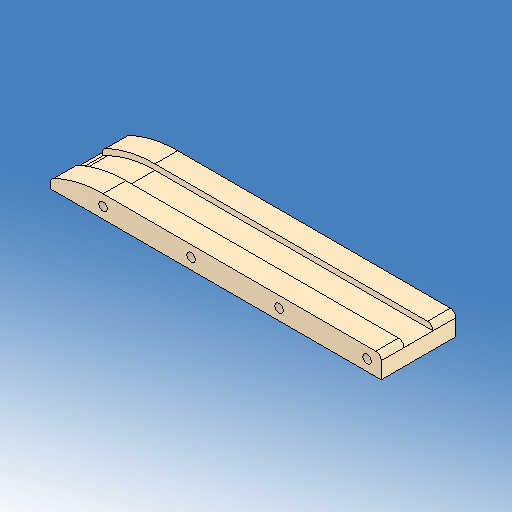
# Autodesk Inventor part: chain guide
Saved by Autodesk Inventor 2025 (Build 290162000, 162)
## iProperties
Created: 2023-03-01
Part Number: chain guide
Material: Polyethylene, High Density
Document SubType Name: Modeling
Designer: ralph
Density: 0.952 g/cm^3
Appearance: Smooth - Off-White
Author: ralph
Autodesk Inventor part; units mm, degrees
(part 1 of 2)
ref_plane "Work Plane1" through (161.724971, -21.836185, 0) normal (0, 0, 1) x (-0.4541702, 0.8909149, 0)
ref_plane "Work Plane2" through (-185.342071, -221.252054, 43.0784) normal (0, 0, -1) x (-0.1993348, 0.9799314, 0)
sketch "Sketch1" plane through (161.724971, -21.836185, 0) normal (0, 0, 1) x (-0.4541702, 0.8909149, 0)
  circle A0 centre (-25.19799, 87.680503) radius 3.175
  line L0 (-137.960154, 56.932811) -> (35.815717, 235.351647)
  line L1 (82.547855, 91.780244) -> (42.733083, 68.543644)
  line L2 (134.381301, 156.187054) -> (107.829785, 115.760327)
  line L3 (-111.140721, 21.588661) -> (-101.506151, 29.862833)
  line L4 (-105.643304, 34.680133) -> (-115.277874, 26.405961)
  line L5 (-3.594311, 192.040273) -> (-4.303422, 192.730924)
  line L6 (-3.594311, 192.040273) -> (-10.222625, 185.234864)
  line L7 (-10.931735, 185.925514) -> (-10.222625, 185.234864)
  arc A1 (2.942016, 134.774843) -> (-78.867042, 82.739265) centre (-35.469099, 104.836969) ccw
  line L8 (2.942016, 134.774843) -> (32.675099, 96.626481)
  arc A2 (44.414913, 71.120558) -> (32.675099, 96.626481) centre (-15.752877, 58.8814) ccw
  line L9 (44.414913, 71.120558) -> (83.682207, -121.91774)
  arc A3 (34.145903, -139.208204) -> (83.682207, -121.91774) centre (57.738523, -127.19513) ccw
  line L10 (34.145903, -139.208204) -> (-78.867042, 82.739265)
  line L11 (86.79349, -121.284852) -> (47.526196, 71.753446)
  arc A4 (47.526196, 71.753446) -> (35.179314, 98.578283) centre (-15.752877, 58.8814) ccw
  line L12 (35.179314, 98.578283) -> (5.446231, 136.726645)
  arc A5 (5.446231, 136.726645) -> (-81.696374, 81.298604) centre (-35.469099, 104.836969) ccw
  line L13 (-81.696374, 81.298604) -> (31.316571, -140.648865)
  arc A6 (31.316571, -140.648865) -> (86.79349, -121.284852) centre (57.738523, -127.19513) ccw
  line L14 (74.34836, -123.816404) -> (35.081066, 69.221894)
  arc A7 (35.081066, 69.221894) -> (25.162453, 90.771076) centre (-15.752877, 58.8814) ccw
  line L15 (25.162453, 90.771076) -> (-4.57063, 128.919438)
  arc A8 (-4.57063, 128.919438) -> (-70.379046, 87.061249) centre (-35.469099, 104.836969) ccw
  line L16 (-70.379046, 87.061249) -> (42.6339, -134.88622)
  arc A9 (42.6339, -134.88622) -> (74.34836, -123.816404) centre (57.738523, -127.19513) ccw
  arc A10 (5.840596, 137.034015) -> (-82.141938, 81.071728) centre (-35.469099, 104.836969) ccw
  line L17 (5.840596, 137.034015) -> (35.573679, 98.885654)
  arc A11 (48.016161, 71.853114) -> (35.573679, 98.885654) centre (-15.752877, 58.8814) ccw
  line L18 (48.016161, 71.853114) -> (87.283455, -121.185185)
  arc A12 (30.871007, -140.875741) -> (87.283455, -121.185185) centre (57.738523, -127.19513) ccw
  line L19 (30.871007, -140.875741) -> (-82.141938, 81.071728)
  line L20 (35.081066, 69.221894) -> (26.965843, 109.116392)
  circle A13 centre (57.738523, -127.19513) radius 44.45
  line L21 (76.564874, -86.928878) -> (65.823198, -81.906643)
  line L22 (5.091971, 163.504868) -> (21.707035, 97.430996)
  line L23 (16.959788, 93.955303) -> (-30.179917, 123.063587)
  line L24 (-32.869192, 137.518787) -> (-4.591446, 166.552061)
  line L25 (29.816468, 96.427864) -> (15.424243, 153.662068)
  line L26 (20.79343, 156.635425) -> (60.850023, 114.922703)
  line L27 (59.720131, 100.498003) -> (42.266373, 90.311684)
  line L28 (16.752459, 188.466235) -> (29.554478, 201.6103)
  line L29 (102.791645, 142.788647) -> (91.891787, 126.192776)
  line L30 (66.346153, 120.200561) -> (40.797068, 146.805966)
  line L31 (-106.606458, 61.811399) -> (-103.834749, 64.657164)
  line L32 (-88.173268, 62.778772) -> (-84.305135, 57.816691)
  line L33 (-71.902397, 23.680787) -> (-75.267331, 21.716952)
  line L34 (-82.428573, 45.397297) -> (-80.279259, 47.243129)
  line L35 (-75.706636, 46.78645) -> (-69.919657, 39.362855)
  line L36 (41.018546, 151.413723) -> (46.086473, 155.76606)
  line L37 (41.121889, 161.54682) -> (35.464526, 156.688275)
  line L38 (31.105895, 156.897817) -> (17.932591, 170.615767)
  line L39 (-84.740604, 53.45607) -> (-87.393157, 51.178057)
  arc A14 (19.642871, 91.662594) -> (21.445924, 90.856947) centre (24.92977, 101.074326) ccw
  arc A15 (23.578481, 87.516275) -> (21.445924, 90.856947) centre (20.421264, 87.851835) ccw
  arc A16 (23.578481, 87.516275) -> (24.03183, 82.566279) centre (36.191661, 86.175702) ccw
  arc A17 (22.700522, 78.989189) -> (24.03183, 82.566279) centre (20.98809, 81.662801) ccw
  line L40 (22.700522, 78.989189) -> (6.045724, 68.321892)
  arc A18 (2.215102, 68.630362) -> (6.045724, 68.321892) centre (4.333292, 70.995504) ccw
  arc A19 (2.215102, 68.630362) -> (-6.080111, 71.872214) centre (-6.267606, 59.158683) ccw
  arc A20 (-8.905438, 73.693574) -> (-6.080111, 71.872214) centre (-6.033293, 75.046869) ccw
  line L41 (-8.905438, 73.693574) -> (-12.804922, 81.969586)
  arc A21 (-12.985819, 84.194406) -> (-12.804922, 81.969586) centre (-9.932777, 83.322881) ccw
  arc A22 (-12.985819, 84.194406) -> (-20.111454, 99.31739) centre (-25.19799, 87.680503) ccw
  arc A23 (-21.711965, 100.873317) -> (-20.111454, 99.31739) centre (-18.839819, 102.226612) ccw
  line L42 (-21.711965, 100.873317) -> (-28.578282, 115.445944)
  arc A24 (-26.364724, 117.50667) -> (-28.578282, 115.445944) centre (-27.142209, 116.122592) ccw
  line L43 (-26.364724, 117.50667) -> (19.642871, 91.662594)
  line L44 (-65.60794, 77.010503) -> (-80.772151, 80.874337)
  line L45 (-82.490843, 86.571338) -> (-54.213097, 115.604612)
  line L46 (-42.284096, 112.695685) -> (-42.24754, 112.608973)
  line L47 (-99.979245, 13.668511) -> (-98.035437, 10.337963)
  line L48 (118.443303, 166.619502) -> (116.943486, 164.335916)
  line L49 (-124.328477, 43.615881) -> (-123.070102, 44.907878)
  line L50 (-120.825239, 44.937466) -> (-116.194419, 40.427197)
  line L51 (-43.104595, 108.966969) -> (-65.061673, 90.110222)
  line L52 (-65.401739, 85.633029) -> (-62.415382, 82.155716)
  ellipse E0 centre (81.305166, 191.046395) end of major axis (135.808144, 158.463034) minor radius 63.499313 (134.381301, 156.187054) -> (35.815717, 235.351647) ccw
  ellipse E1 centre (44.138423, 157.591537) end of major axis (-21.265151, 196.691569) minor radius 76.199176 (82.547855, 91.780244) -> (107.829785, 115.760327) ccw
  ellipse E2 centre (-113.209297, 23.997311) end of major axis (-115.934446, 25.626479) minor radius 3.174966 (-115.277874, 26.405961) -> (-111.140721, 21.588661) ccw
  ellipse E3 centre (-103.574727, 32.271483) end of major axis (-106.299876, 33.900651) minor radius 3.174966 (-101.506151, 29.862833) -> (-105.643304, 34.680133) ccw
  ellipse E4 centre (5.31041, 178.259198) end of major axis (-5.590186, 184.77587) minor radius 12.699863 (-0.791497, 167.121278) -> (2.672353, 165.836334) ccw
  ellipse E5 centre (2.012839, 162.730619) end of major axis (-0.71231, 164.359787) minor radius 3.174966 (5.091971, 163.504868) -> (2.672353, 165.836334) ccw
  ellipse E6 centre (18.627903, 96.656747) end of major axis (21.353052, 95.027579) minor radius 3.174966 (16.959788, 93.955303) -> (21.707035, 97.430996) ccw
  ellipse E7 centre (-28.511802, 125.76503) end of major axis (-25.786653, 124.135862) minor radius 3.174966 (-31.67169, 126.074374) -> (-30.179917, 123.063587) ccw
  ellipse E8 centre (-44.311242, 127.311749) end of major axis (-55.211837, 133.828421) minor radius 12.699863 (-31.67169, 126.074374) -> (-33.338024, 133.705169) ccw
  ellipse E9 centre (-30.59472, 135.303524) end of major axis (-27.869571, 133.674356) minor radius 3.174966 (-32.869192, 137.518787) -> (-33.338024, 133.705169) ccw
  ellipse E10 centre (-2.316974, 164.336798) end of major axis (-5.042123, 165.965966) minor radius 3.174966 (-0.791497, 167.121278) -> (-4.591446, 166.552061) ccw
  ellipse E11 centre (32.8956, 97.202113) end of major axis (35.620749, 95.572945) minor radius 3.174966 (29.816468, 96.427864) -> (32.236086, 94.096397) ccw
  ellipse E12 centre (18.503375, 154.436317) end of major axis (15.778226, 156.065485) minor radius 3.174966 (20.79343, 156.635425) -> (15.424243, 153.662068) ccw
  ellipse E13 centre (58.559969, 112.723596) end of major axis (55.83482, 114.352764) minor radius 3.174966 (61.542416, 111.634731) -> (60.850023, 114.922703) ccw
  ellipse E14 centre (73.472205, 107.279273) end of major axis (62.571609, 113.795945) minor radius 12.699863 (61.542416, 111.634731) -> (61.190231, 104.047967) ccw
  ellipse E15 centre (58.119738, 103.240141) end of major axis (60.844887, 101.610973) minor radius 3.174966 (59.720131, 100.498003) -> (61.190231, 104.047967) ccw
  ellipse E16 centre (40.66598, 93.053821) end of major axis (43.391128, 91.424653) minor radius 3.174966 (38.452389, 90.777764) -> (42.266373, 90.311684) ccw
  ellipse E17 centre (20.222646, 172.814875) end of major axis (22.947795, 171.185707) minor radius 3.174966 (17.240198, 173.903739) -> (17.932591, 170.615767) ccw
  ellipse E18 centre (5.31041, 178.259198) end of major axis (-5.590186, 184.77587) minor radius 12.699863 (17.240198, 173.903739) -> (16.283627, 184.652618) ccw
  ellipse E19 centre (19.026932, 186.250973) end of major axis (21.752081, 184.621805) minor radius 3.174966 (16.752459, 188.466235) -> (16.283627, 184.652618) ccw
  ellipse E20 centre (31.82895, 199.395037) end of major axis (29.103801, 201.024205) minor radius 3.174966 (34.959397, 198.865037) -> (29.554478, 201.6103) ccw
  ellipse E21 centre (81.290008, 191.021041) end of major axis (40.957805, 215.132728) minor radius 46.989492 (50.252199, 155.741184) -> (98.944937, 147.473983) ccw
  ellipse E22 centre (100.137838, 144.531614) end of major axis (97.412689, 146.160782) minor radius 3.174966 (102.791645, 142.788647) -> (98.944937, 147.473983) ccw
  ellipse E23 centre (44.123265, 157.566183) end of major axis (-4.929415, 186.891207) minor radius 57.149382 (85.199308, 117.83109) -> (91.891787, 126.192776) ccw
  ellipse E24 centre (82.917305, 120.038595) end of major axis (85.642454, 118.409427) minor radius 3.174966 (81.028285, 117.486731) -> (85.199308, 117.83109) ccw
  ellipse E25 centre (73.472205, 107.279273) end of major axis (62.571609, 113.795945) minor radius 12.699863 (81.028285, 117.486731) -> (69.603407, 119.37559) ccw
  ellipse E26 centre (68.636207, 122.399669) end of major axis (71.361356, 120.770501) minor radius 3.174966 (66.346153, 120.200561) -> (69.603407, 119.37559) ccw
  ellipse E27 centre (-108.40717, 28.109043) end of major axis (-132.93351, 42.771555) minor radius 28.574691 (-80.021668, 24.824085) -> (-83.164714, 41.500687) ccw
  ellipse E28 centre (-104.331986, 59.596136) end of major axis (-101.606837, 57.966968) minor radius 3.174966 (-106.606458, 61.811399) -> (-104.739504, 56.447427) ccw
  ellipse E29 centre (-101.560276, 62.441901) end of major axis (-104.285425, 64.071069) minor radius 3.174966 (-100.034799, 65.226381) -> (-103.834749, 64.657164) ccw
  ellipse E30 centre (-93.932893, 76.3643) end of major axis (-83.032297, 69.847628) minor radius 12.699863 (-100.034799, 65.226381) -> (-91.32843, 63.934301) ccw
  ellipse E31 centre (-90.677314, 60.826801) end of major axis (-93.402463, 62.455969) minor radius 3.174966 (-88.173268, 62.778772) -> (-91.32843, 63.934301) ccw
  ellipse E32 centre (-72.423703, 37.410884) end of major axis (-75.148852, 39.040052) minor radius 3.174966 (-69.569027, 36.021118) -> (-69.919657, 39.362855) ccw
  ellipse E33 centre (-58.150322, 30.462056) end of major axis (-69.050918, 36.978728) minor radius 12.699863 (-69.569027, 36.021118) -> (-70.432296, 27.23075) ccw
  ellipse E34 centre (-73.50279, 26.422924) end of major axis (-70.777641, 24.793756) minor radius 3.174966 (-71.902397, 23.680787) -> (-70.432296, 27.23075) ccw
  ellipse E35 centre (-76.867724, 24.459089) end of major axis (-74.142575, 22.829921) minor radius 3.174966 (-80.021668, 24.824085) -> (-75.267331, 21.716952) ccw
  ellipse E36 centre (-108.40717, 28.109043) end of major axis (-132.93351, 42.771555) minor radius 28.574691 (-91.356277, 51.038941) -> (-104.739504, 56.447427) ccw
  ellipse E37 centre (81.290008, 191.021041) end of major axis (40.957805, 215.132728) minor radius 46.989492 (34.959397, 198.865037) -> (41.726521, 165.668481) ccw
  ellipse E38 centre (-80.359997, 42.988647) end of major axis (-83.085146, 44.617815) minor radius 3.174966 (-82.428573, 45.397297) -> (-83.164714, 41.500687) ccw
  ellipse E39 centre (-78.210682, 44.834479) end of major axis (-80.935831, 46.463647) minor radius 3.174966 (-75.706636, 46.78645) -> (-80.279259, 47.243129) ccw
  ellipse E40 centre (43.087122, 149.005073) end of major axis (45.812271, 147.375905) minor radius 3.174966 (41.018546, 151.413723) -> (40.797068, 146.805966) ccw
  ellipse E41 centre (48.155049, 153.35741) end of major axis (45.4299, 154.986578) minor radius 3.174966 (50.252199, 155.741184) -> (46.086473, 155.76606) ccw
  ellipse E42 centre (33.39595, 159.096925) end of major axis (36.121098, 157.467757) minor radius 3.174966 (31.105895, 156.897817) -> (35.464526, 156.688275) ccw
  ellipse E43 centre (39.053313, 163.95547) end of major axis (36.328164, 165.584638) minor radius 3.174966 (41.121889, 161.54682) -> (41.726521, 165.668481) ccw
  ellipse E44 centre (-86.80918, 55.86472) end of major axis (-89.534329, 57.493888) minor radius 3.174966 (-84.740604, 53.45607) -> (-84.305135, 57.816691) ccw
  ellipse E45 centre (-89.461733, 53.586707) end of major axis (-86.736584, 51.957539) minor radius 3.174966 (-91.356277, 51.038941) -> (-87.393157, 51.178057) ccw
  ellipse E46 centre (-79.988236, 83.951008) end of major axis (-77.263087, 82.32184) minor radius 3.174966 (-82.777167, 82.433666) -> (-80.772151, 80.874337) ccw
  ellipse E47 centre (-93.932893, 76.3643) end of major axis (-104.833488, 82.880972) minor radius 12.699863 (-82.777167, 82.433666) -> (-82.959675, 82.75772) ccw
  ellipse E48 centre (-80.216371, 84.356075) end of major axis (-77.491222, 82.726907) minor radius 3.174966 (-82.490843, 86.571338) -> (-82.959675, 82.75772) ccw
  ellipse E49 centre (-51.938625, 113.38935) end of major axis (-54.663774, 115.018518) minor radius 3.174966 (-50.413148, 116.173829) -> (-54.213097, 115.604612) ccw
  ellipse E50 centre (-44.311242, 127.311749) end of major axis (-33.410646, 120.795077) minor radius 12.699863 (-50.413148, 116.173829) -> (-45.03003, 114.632214) ccw
  ellipse E51 centre (-45.209727, 111.46233) end of major axis (-47.934876, 113.091498) minor radius 3.174966 (-42.284096, 112.695685) -> (-45.03003, 114.632214) ccw
  ellipse E52 centre (69.174216, 230.477557) end of major axis (66.449067, 232.106725) minor radius 3.174966 (71.822052, 228.725533) -> (68.242232, 233.512673) ccw
  ellipse E53 centre (87.709071, 218.213391) end of major axis (71.358177, 227.988399) minor radius 19.049794 (71.822052, 228.725533) -> (69.767585, 224.616929) ccw
  ellipse E54 centre (66.777338, 225.684185) end of major axis (69.502486, 224.055017) minor radius 3.174966 (65.439426, 222.80488) -> (69.767585, 224.616929) ccw
  ellipse E55 centre (57.411955, 205.529045) end of major axis (41.061062, 215.304053) minor radius 19.049794 (65.439426, 222.80488) -> (61.070524, 224.224243) ccw
  ellipse E56 centre (61.680285, 227.340109) end of major axis (64.405434, 225.710941) minor radius 3.174966 (60.171845, 230.133884) -> (61.070524, 224.224243) ccw
  ellipse E57 centre (81.290008, 191.021041) end of major axis (119.442093, 168.212688) minor radius 44.449519 (68.242232, 233.512673) -> (60.171845, 230.133884) ccw
  ellipse E58 centre (115.071482, 214.736161) end of major axis (117.796631, 213.106993) minor radius 3.174966 (114.22345, 211.676543) -> (117.670057, 216.560401) ccw
  ellipse E59 centre (109.13526, 193.318833) end of major axis (92.784366, 203.093841) minor radius 19.049794 (114.22345, 211.676543) -> (109.681031, 212.360856) ccw
  ellipse E60 centre (109.771993, 215.534527) end of major axis (112.497142, 213.905359) minor radius 3.174966 (106.620147, 215.917221) -> (109.681031, 212.360856) ccw
  ellipse E61 centre (87.709071, 218.213391) end of major axis (71.358177, 227.988399) minor radius 19.049794 (106.620147, 215.917221) -> (106.619944, 220.510867) ccw
  ellipse E62 centre (109.771757, 220.89378) end of major axis (107.046608, 222.522948) minor radius 3.174966 (111.96266, 223.191683) -> (106.619944, 220.510867) ccw
  ellipse E63 centre (81.290008, 191.021041) end of major axis (119.442093, 168.212688) minor radius 44.449519 (117.670057, 216.560401) -> (111.96266, 223.191683) ccw
  ellipse E64 centre (-99.406505, 9.537784) end of major axis (-98.043931, 8.7232) minor radius 1.587483 (-98.714147, 8.109225) -> (-98.035437, 10.337963) ccw
  ellipse E65 centre (-108.40717, 28.109043) end of major axis (-127.483212, 39.513219) minor radius 22.22476 (-107.641506, 5.897406) -> (-98.714147, 8.109225) ccw
  ellipse E66 centre (-107.750887, 9.070497) end of major axis (-110.476036, 10.699665) minor radius 3.174966 (-108.8456, 12.050789) -> (-107.641506, 5.897406) ccw
  ellipse E67 centre (-113.224455, 23.971957) end of major axis (-102.323859, 17.455285) minor radius 12.699863 (-108.8456, 12.050789) -> (-104.821996, 14.448914) ccw
  ellipse E68 centre (-102.721381, 12.068153) end of major axis (-99.996232, 10.438985) minor radius 3.174966 (-99.979245, 13.668511) -> (-104.821996, 14.448914) ccw
  ellipse E69 centre (114.28968, 166.078883) end of major axis (117.014829, 164.449715) minor radius 3.174966 (111.116905, 165.9603) -> (116.943486, 164.335916) ccw
  ellipse E70 centre (92.080258, 165.248804) end of major axis (75.729364, 175.023813) minor radius 19.049794 (111.116905, 165.9603) -> (110.359048, 170.613884) ccw
  ellipse E71 centre (113.405514, 171.508064) end of major axis (110.680365, 173.137232) minor radius 3.174966 (112.795477, 174.623888) -> (110.359048, 170.613884) ccw
  ellipse E72 centre (109.13526, 193.318833) end of major axis (92.784366, 203.093841) minor radius 19.049794 (112.795477, 174.623888) -> (117.164254, 176.043554) ccw
  ellipse E73 centre (118.50242, 173.16434) end of major axis (115.777271, 174.793508) minor radius 3.174966 (121.364913, 171.790748) -> (117.164254, 176.043554) ccw
  ellipse E74 centre (81.290008, 191.021041) end of major axis (119.442093, 168.212688) minor radius 44.449519 (118.443303, 166.619502) -> (121.364913, 171.790748) ccw
  ellipse E75 centre (-121.932866, 43.800246) end of major axis (-123.29544, 44.61483) minor radius 1.587483 (-120.825239, 44.937466) -> (-123.070102, 44.907878) ccw
  ellipse E76 centre (-117.302045, 39.289977) end of major axis (-118.66462, 40.104561) minor radius 1.587483 (-116.313726, 38.047651) -> (-116.194419, 40.427197) ccw
  ellipse E77 centre (-108.40717, 28.109043) end of major axis (-119.307765, 34.625715) minor radius 12.699863 (-116.313726, 38.047651) -> (-118.827374, 35.369161) ccw
  ellipse E78 centre (-113.224455, 23.971957) end of major axis (-102.323859, 17.455285) minor radius 12.699863 (-118.827374, 35.369161) -> (-124.347508, 30.101205) ccw
  ellipse E79 centre (-127.128271, 31.633517) end of major axis (-129.85342, 33.262685) minor radius 3.174966 (-130.248455, 32.22093) -> (-124.347508, 30.101205) ccw
  ellipse E80 centre (-108.40717, 28.109043) end of major axis (-127.483212, 39.513219) minor radius 22.22476 (-124.328477, 43.615881) -> (-130.248455, 32.22093) ccw
  ellipse E81 centre (29.598029, 81.673534) end of major axis (18.697433, 88.190206) minor radius 12.699863 (38.452389, 90.777764) -> (32.236086, 94.096397) ccw
  ellipse E82 centre (-62.993097, 87.701572) end of major axis (-60.267948, 86.072404) minor radius 3.174966 (-65.061673, 90.110222) -> (-65.401739, 85.633029) ccw
  ellipse E83 centre (-64.824025, 80.087173) end of major axis (-62.098876, 78.458005) minor radius 3.174966 (-65.60794, 77.010503) -> (-62.415382, 82.155716) ccw
  ellipse E84 centre (-48.97507, 61.632654) end of major axis (-51.700218, 63.261822) minor radius 3.174966 (-46.566427, 63.701197) -> (-48.191155, 64.709325) ccw
  line L53 (-46.566427, 63.701197) -> (-45.046946, 61.931914)
  ellipse E85 centre (-42.638304, 64.000457) end of major axis (-39.913155, 62.371289) minor radius 3.174966 (-45.046946, 61.931914) -> (-40.671405, 61.508088) ccw
  ellipse E86 centre (-38.704505, 59.015719) end of major axis (-35.979357, 57.386551) minor radius 3.174966 (-37.92059, 62.092389) -> (-40.671405, 61.508088) ccw
  line L54 (-37.92059, 62.092389) -> (-29.348807, 59.908302)
  line L55 (-78.860233, 72.523793) -> (-48.191155, 64.709325)
  ellipse E87 centre (2.464984, 188.372176) end of major axis (0.556333, 189.515712) minor radius 2.224976
  ellipse E88 centre (-6.396024, 179.274418) end of major axis (-4.487373, 178.130882) minor radius 2.224976
  ellipse E89 centre (-6.396024, 179.274418) end of major axis (-11.457168, 182.306716) minor radius 5.899936 (-10.825614, 183.171688) -> (-0.62485, 178.04826) ccw
  ellipse E90 centre (5.244141, 176.80132) end of major axis (10.391067, 173.717628) minor radius 5.999935 (3.842886, 182.635365) -> (-0.62485, 178.04826) ccw
  ellipse E91 centre (2.464984, 188.372176) end of major axis (-2.596159, 191.404473) minor radius 5.899936 (3.842886, 182.635365) -> (-1.547741, 192.697448) ccw
  ellipse E92 centre (-2.907987, 194.163641) end of major axis (-4.623629, 195.191539) minor radius 1.999978 (-4.303422, 192.730924) -> (-1.547741, 192.697448) ccw
  ellipse E93 centre (-12.32717, 184.492797) end of major axis (-10.611528, 183.464899) minor radius 1.999978 (-10.825614, 183.171688) -> (-10.931735, 185.925514) ccw
  ellipse E94 centre (-108.392012, 28.134397) end of major axis (-72.965077, 6.955213) minor radius 41.274553 (-137.960154, 56.932811) -> (-87.586903, -7.513386) ccw
  arc A25 (42.733083, 68.543644) -> (42.293157, 68.286896) centre (41.303631, 70.48767) ccw
  circle A26 centre (-43.147851, 88.298968) radius 12.7
  ellipse E95 centre (-45.173171, 111.375619) end of major axis (-47.89832, 113.004787) minor radius 3.174966 (-43.104595, 108.966969) -> (-42.24754, 112.608973) ccw
  ellipse E96 centre (-30.132722, 56.831632) end of major axis (-32.85787, 58.4608) minor radius 3.174966 (-26.961407, 56.678865) -> (-29.348807, 59.908302) ccw
  line L56 (42.293157, 68.286896) -> (-87.586903, -7.513386)
  ellipse E97 centre (-14.276147, 56.067795) end of major axis (-25.176742, 62.584467) minor radius 12.699863 (-26.961407, 56.678865) -> (-26.55812, 52.836489) ccw
  ellipse E98 centre (-29.628614, 52.028663) end of major axis (-26.903465, 50.399495) minor radius 3.174966 (-28.028221, 49.286526) -> (-26.55812, 52.836489) ccw
  line L57 (-28.028221, 49.286526) -> (-45.481979, 39.100206)
  ellipse E99 centre (-47.082372, 41.842343) end of major axis (-44.357223, 40.213175) minor radius 3.174966 (-49.295962, 39.566286) -> (-45.481979, 39.100206) ccw
  ellipse E100 centre (-58.150322, 30.462056) end of major axis (-69.050918, 36.978728) minor radius 12.699863 (-49.295962, 39.566286) -> (-60.754786, 42.892056) ccw
  ellipse E101 centre (-61.405902, 45.999556) end of major axis (-58.680753, 44.370388) minor radius 3.174966 (-63.909947, 44.047585) -> (-60.754786, 42.892056) ccw
  line L58 (-63.909947, 44.047585) -> (-82.163558, 67.463502)
  ellipse E102 centre (-79.659513, 69.415473) end of major axis (-76.934364, 67.786305) minor radius 3.174966 (-82.514189, 70.805238) -> (-82.163558, 67.463502) ccw
  ellipse E103 centre (-93.932893, 76.3643) end of major axis (-83.032297, 69.847628) minor radius 12.699863 (-82.514189, 70.805238) -> (-82.501897, 70.830558) ccw
  ellipse E104 centre (-79.644148, 69.447122) end of major axis (-76.918999, 67.817954) minor radius 3.174966 (-78.860233, 72.523793) -> (-82.501897, 70.830558) ccw
  point P0 (92.904845, 134.165849)
  point P1 (66.157421, -83.549687)
  point P2 (80.192286, -88.833286)
  point P3 (-35.470288, 104.862264)
  point P4 (57.737333, -127.169835)
  dimension "d3" = 88.9
  dimension "d0" = 3.175
  dimension "d2" = 12.7
  constraints: 28 end point, 24 point on circle, 12 centre point, 3 point on line, 1 coincident, 1 collinear, 131 other
  measures "d0" distance between parallel lines of L9 L11
  measures "d2" distance between parallel lines of L11 L14
extrude "Extrusion1" add sketch "Sketch1" along normal up to surface (43.0784 mm away) contours A13 L9 L1 L11 | L56 A25 L1 L9 L21 L14 | L14 L20 L25 E11 E81 A2 L9 L1 A25 L56 | L14 L21 A13 | L1 L9 A2 E81 E16 A4 L11 | L20 L12 A4 E16 E81 A2 L8 | L8 A2 E81 E11 L25 L20
fillet "Fillet1" radius 3.175 1 edges at (52.2645, -47.3693, 21.5392)
ref_plane "Work Plane3" through (204.446927, 89.953752, 21.5392) normal (0, 0, 1) x (-0.622646, 0.7825036, 0)
sketch "Sketch3" plane through (204.446927, 89.953752, 21.5392) normal (0, 0, 1) x (-0.622646, 0.7825036, 0)
  line L0 (-184.738082, 186.304337) -> (21.115446, 326.502981)
  line L1 (38.290956, 176.497506) -> (-148.222121, 113.110339)
  line L2 (101.9227, 229.279553) -> (67.84558, 194.956774)
  line L3 (-168.596067, 151.868749) -> (-157.505518, 158.056364)
  line L4 (-154.411647, 152.511062) -> (-165.502196, 146.323446)
  line L5 (-121.649585, 199.840185) -> (-55.146507, -40.180534)
  arc A0 (-55.146507, -40.180534) -> (-3.192917, -33.116159) centre (-29.65, -33.116159) ccw
  line L6 (-3.192917, -33.116159) -> (-3.192917, 163.875478)
  arc A1 (-3.192917, 163.875478) -> (-9.611038, 191.201711) centre (-64.575, 163.875478) ccw
  line L7 (-9.611038, 191.201711) -> (-31.143124, 234.511329)
  arc A2 (-31.143124, 234.511329) -> (-121.649585, 199.840185) centre (-74.735, 212.838914) ccw
  line L8 (-125.18879, 198.85957) -> (-58.685712, -41.161149)
  arc A3 (-58.685712, -41.161149) -> (0.479628, -33.116159) centre (-29.65, -33.116159) ccw
  line L9 (0.479628, -33.116159) -> (0.479628, 163.875478)
  arc A4 (0.479628, 163.875478) -> (-6.322496, 192.836664) centre (-64.575, 163.875478) ccw
  line L10 (-6.322496, 192.836664) -> (-27.854582, 236.146282)
  arc A5 (-27.854582, 236.146282) -> (-125.18879, 198.85957) centre (-74.735, 212.838914) ccw
  line L11 (0, 0) -> (0, 163.875478)
  arc A6 (0, 0) -> (-12.7, 7.975202) centre (-29.65, -33.116159) ccw
  arc A7 (0, 163.875478) -> (-6.678359, 192.474597) centre (-64.575, 163.875478) ccw
  arc A8 (-6.678359, 192.474597) -> (-12.7, 191.068446) centre (-9.525, 191.068446) ccw
  line L12 (-12.7, 191.068446) -> (-12.7, 7.975202)
  line L13 (0, 0) -> (-3.192917, 2.268858)
  line L14 (-3.192917, 2.602537) -> (-3.192917, 163.875478)
  line L15 (-65.672645, 244.346603) -> (-32.17505, 267.160482)
  line L16 (-126.614388, 140.573845) -> (-130.303253, 139.32017)
  line L17 (-153.02123, 184.856959) -> (-149.737884, 187.093115)
  line L18 (68.316141, 222.468776) -> (54.326892, 208.37868)
  line L19 (17.679011, 189.612497) -> (-1.454963, 183.109744)
  line L20 (-30.418788, 173.26628) -> (-49.552763, 166.763527)
  line L21 (-123.696478, 189.823582) -> (-95.20058, 176.052523)
  line L22 (-78.516588, 156.920062) -> (-97.650563, 150.417309)
  line L23 (-114.722523, 158.938737) -> (-127.942203, 185.523311)
  line L24 (-65.592841, 218.887637) -> (-28.591878, 184.149965)
  line L25 (-62.761728, 175.550795) -> (-64.149554, 182.45772)
  line L26 (-69.358845, 208.383293) -> (-70.87874, 215.947497)
  line L27 (-79.846714, 221.898384) -> (-79.828176, 221.806125)
  line L28 (-109.815782, 191.578606) -> (-123.905473, 198.387654)
  line L29 (-124.454062, 204.31292) -> (-90.956467, 227.126798)
  line L30 (-134.765136, 182.130541) -> (-131.963746, 176.496989)
  line L31 (28.099465, 207.598856) -> (8.366497, 238.76315)
  line L32 (-12.435848, 191.584881) -> (-15.130471, 250.539349)
  line L33 (-9.276344, 252.382768) -> (21.661574, 203.522487)
  line L34 (-23.293378, 262.244199) -> (-20.182577, 194.184374)
  line L35 (-25.52738, 191.724725) -> (-65.918765, 229.645432)
  line L36 (-133.2597, 172.310683) -> (-136.313107, 170.607133)
  line L37 (0.88147, 250.584261) -> (-9.293, 266.65281)
  line L38 (11.623165, 253.143429) -> (5.11086, 249.510097)
  line L39 (-132.600462, 163.95277) -> (-130.126343, 165.333126)
  line L40 (-125.736518, 163.974129) -> (-121.545457, 155.545967)
  line L41 (9.502017, 243.234289) -> (15.33581, 246.489066)
  line L42 (-174.014593, 170.559215) -> (-172.523932, 171.574445)
  line L43 (-170.318223, 171.15596) -> (-166.679391, 165.813122)
  line L44 (-156.123569, 136.359195) -> (-154.882666, 132.708018)
  line L45 (88.404012, 242.701459) -> (86.479096, 240.762666)
  line L46 (-81.39401, 218.408051) -> (-106.669248, 204.306543)
  line L47 (-107.89495, 199.986988) -> (-105.661674, 195.984174)
  line L48 (-85.657777, 171.440825) -> (-77.693381, 167.591914)
  line L49 (-93.809413, 174.740762) -> (-92.673106, 172.704101)
  line L50 (-59.845082, 191.019444) -> (-69.018713, 207.461812)
  line L51 (-62.583721, 185.855794) -> (-61.070784, 186.699889)
  ellipse E0 centre (0.081872, 301.433332) end of major axis (-4.251088, 305.437762) minor radius 5.899933 (0.288576, 295.536988) -> (-2.988147, 306.471677) ccw
  ellipse E1 centre (0.077895, 301.429029) end of major axis (1.711935, 299.918884) minor radius 2.224975
  ellipse E2 centre (-161.503857, 152.189905) end of major axis (-131.009638, 124.373935) minor radius 41.274553 (-184.738082, 186.304337) -> (-148.222121, 113.110339) ccw
  ellipse E3 centre (13.770828, 248.644398) end of major axis (-42.526191, 299.99696) minor radius 76.199176 (38.290956, 176.497506) -> (67.84558, 194.956774) ccw
  ellipse E4 centre (56.860407, 274.019239) end of major axis (103.77459, 231.225438) minor radius 63.499313 (101.9227, 229.279553) -> (21.115446, 326.502981) ccw
  ellipse E5 centre (-155.958582, 155.283713) end of major axis (-158.304292, 157.423403) minor radius 3.174966 (-154.411647, 152.511062) -> (-157.505518, 158.056364) ccw
  ellipse E6 centre (-167.049131, 149.096097) end of major axis (-169.39484, 151.235788) minor radius 3.174966 (-168.596067, 151.868749) -> (-165.502196, 146.323446) ccw
  ellipse E7 centre (-137.701105, 196.591521) end of major axis (-147.083941, 205.150282) minor radius 12.699863 (-145.90073, 186.893446) -> (-137.626641, 183.891814) ccw
  ellipse E8 centre (-111.786555, 144.477757) end of major axis (-102.403718, 135.918997) minor radius 12.699863 (-101.295099, 151.634295) -> (-111.861018, 157.177464) ccw
  ellipse E9 centre (-127.63606, 143.579966) end of major axis (-125.290351, 141.440275) minor radius 3.174966 (-126.614388, 140.573845) -> (-124.466159, 143.759524) ccw
  ellipse E10 centre (-131.324925, 142.326291) end of major axis (-128.979216, 140.186601) minor radius 3.174966 (-134.342818, 143.312652) -> (-130.303253, 139.32017) ccw
  ellipse E11 centre (-151.233982, 182.232772) end of major axis (-148.888273, 180.093082) minor radius 3.174966 (-153.02123, 184.856959) -> (-152.260969, 179.228485) ccw
  ellipse E12 centre (-147.950636, 184.468928) end of major axis (-150.296346, 186.608618) minor radius 3.174966 (-145.90073, 186.893446) -> (-149.737884, 187.093115) ccw
  ellipse E13 centre (-78.919688, 236.625205) end of major axis (-69.536851, 228.066445) minor radius 12.699863 (-66.780445, 232.89316) -> (-66.892255, 240.702974) ccw
  ellipse E14 centre (-63.885397, 241.722416) end of major axis (-61.539688, 239.582726) minor radius 3.174966 (-65.672645, 244.346603) -> (-66.892255, 240.702974) ccw
  ellipse E15 centre (-30.387802, 264.536295) end of major axis (-32.733511, 266.675985) minor radius 3.174966 (-28.337896, 266.960813) -> (-32.17505, 267.160482) ccw
  ellipse E16 centre (-20.138271, 276.658888) end of major axis (-10.755434, 268.100128) minor radius 12.699863 (-28.337896, 266.960813) -> (-25.199695, 265.011191) ccw
  ellipse E17 centre (56.860407, 274.019239) end of major axis (91.576902, 242.351827) minor radius 46.989492 (19.412977, 245.634315) -> (65.480582, 227.826866) ccw
  ellipse E18 centre (66.063026, 224.70576) end of major axis (63.717317, 226.84545) minor radius 3.174966 (68.316141, 222.468776) -> (65.480582, 227.826866) ccw
  ellipse E19 centre (13.770828, 248.644398) end of major axis (-28.451936, 287.15882) minor radius 57.149382 (46.101946, 201.518846) -> (54.326892, 208.37868) ccw
  ellipse E20 centre (44.305773, 204.136932) end of major axis (46.651482, 201.997242) minor radius 3.174966 (41.945987, 202.012828) -> (46.101946, 201.518846) ccw
  ellipse E21 centre (32.506845, 193.516409) end of major axis (41.889681, 184.957649) minor radius 12.699863 (21.684664, 200.162482) -> (19.827241, 192.798176) ccw
  ellipse E22 centre (16.65734, 192.618617) end of major axis (19.003049, 190.478927) minor radius 3.174966 (17.679011, 189.612497) -> (19.827241, 192.798176) ccw
  ellipse E23 centre (-2.476635, 186.115865) end of major axis (-0.130926, 183.976175) minor radius 3.174966 (-5.099499, 184.32673) -> (-1.454963, 183.109744) ccw
  ellipse E24 centre (-15.590955, 177.170192) end of major axis (-6.208119, 168.611431) minor radius 12.699863 (-5.099499, 184.32673) -> (-10.529531, 188.817889) ccw
  ellipse E25 centre (-31.44046, 176.2724) end of major axis (-29.094751, 174.13271) minor radius 3.174966 (-30.418788, 173.26628) -> (-28.270559, 176.451958) ccw
  ellipse E26 centre (-50.574435, 169.769647) end of major axis (-48.228726, 167.629957) minor radius 3.174966 (-53.197299, 167.980513) -> (-49.552763, 166.763527) ccw
  ellipse E27 centre (-79.074852, 164.73325) end of major axis (-81.420561, 166.87294) minor radius 3.174966 (-75.997633, 163.951394) -> (-77.693381, 167.591914) ccw
  ellipse E28 centre (-63.688755, 160.823974) end of major axis (-54.305918, 152.265214) minor radius 12.699863 (-75.997633, 163.951394) -> (-76.368359, 160.105741) ccw
  ellipse E29 centre (-79.53826, 159.926183) end of major axis (-77.192551, 157.786493) minor radius 3.174966 (-78.516588, 156.920062) -> (-76.368359, 160.105741) ccw
  ellipse E30 centre (-98.672235, 153.42343) end of major axis (-96.326525, 151.28374) minor radius 3.174966 (-101.295099, 151.634295) -> (-97.650563, 150.417309) ccw
  ellipse E31 centre (-111.879634, 160.352391) end of major axis (-109.533925, 158.212701) minor radius 3.174966 (-114.722523, 158.938737) -> (-111.861018, 157.177464) ccw
  ellipse E32 centre (-63.688755, 160.823974) end of major axis (-54.305918, 152.265214) minor radius 12.699863 (-53.197299, 167.980513) -> (-60.456919, 173.105769) ccw
  ellipse E33 centre (-59.64896, 176.176218) end of major axis (-57.303251, 174.036528) minor radius 3.174966 (-62.761728, 175.550795) -> (-60.456919, 173.105769) ccw
  ellipse E34 centre (-67.765971, 216.57292) end of major axis (-70.11168, 218.71261) minor radius 3.174966 (-65.592841, 218.887637) -> (-70.87874, 215.947497) ccw
  ellipse E35 centre (-122.524002, 201.246319) end of major axis (-120.178293, 199.106629) minor radius 3.174966 (-125.559423, 200.315359) -> (-123.905473, 198.387654) ccw
  ellipse E36 centre (-137.701105, 196.591521) end of major axis (-128.318268, 188.032761) minor radius 12.699863 (-125.559423, 200.315359) -> (-125.673672, 200.66929) ccw
  ellipse E37 centre (-122.666814, 201.688733) end of major axis (-120.321105, 199.549042) minor radius 3.174966 (-124.454062, 204.31292) -> (-125.673672, 200.66929) ccw
  ellipse E38 centre (-89.169219, 224.502611) end of major axis (-91.514928, 226.642301) minor radius 3.174966 (-87.119313, 226.92713) -> (-90.956467, 227.126798) ccw
  ellipse E39 centre (-78.919688, 236.625205) end of major axis (-88.302524, 245.183965) minor radius 12.699863 (-87.119313, 226.92713) -> (-82.151524, 224.34341) ccw
  ellipse E40 centre (-82.959483, 221.272961) end of major axis (-85.305192, 223.412651) minor radius 3.174966 (-79.846714, 221.898384) -> (-82.151524, 224.34341) ccw
  ellipse E41 centre (-111.786555, 144.477757) end of major axis (-102.403718, 135.918997) minor radius 12.699863 (-121.867987, 152.201402) -> (-124.466159, 143.759524) ccw
  ellipse E42 centre (-137.608025, 180.716887) end of major axis (-139.953734, 182.856577) minor radius 3.174966 (-134.765136, 182.130541) -> (-137.626641, 183.891814) ccw
  ellipse E43 centre (-124.388346, 154.132313) end of major axis (-126.734055, 156.272003) minor radius 3.174966 (-121.867987, 152.201402) -> (-121.545457, 155.545967) ccw
  ellipse E44 centre (-6.610545, 268.351297) end of major axis (-4.264836, 266.211607) minor radius 3.174966 (-9.31609, 270.012816) -> (-9.293, 266.65281) ccw
  ellipse E45 centre (30.78192, 209.297343) end of major axis (33.127629, 207.157653) minor radius 3.174966 (28.099465, 207.598856) -> (31.126905, 206.141156) ccw
  ellipse E46 centre (-9.264175, 191.729814) end of major axis (-6.918466, 189.590124) minor radius 3.174966 (-12.435848, 191.584881) -> (-10.529531, 188.817889) ccw
  ellipse E47 centre (-11.958798, 250.684281) end of major axis (-14.304508, 252.823971) minor radius 3.174966 (-9.276344, 252.382768) -> (-15.130471, 250.539349) ccw
  ellipse E48 centre (18.979119, 201.824) end of major axis (16.63341, 203.96369) minor radius 3.174966 (21.684664, 200.162482) -> (21.661574, 203.522487) ccw
  ellipse E49 centre (-26.465051, 262.099266) end of major axis (-28.81076, 264.238956) minor radius 3.174966 (-23.293378, 262.244199) -> (-25.199695, 265.011191) ccw
  ellipse E50 centre (-23.35425, 194.039441) end of major axis (-21.008541, 191.899751) minor radius 3.174966 (-25.52738, 191.724725) -> (-20.182577, 194.184374) ccw
  ellipse E51 centre (-63.745635, 231.960148) end of major axis (-61.399926, 229.820458) minor radius 3.174966 (-66.780445, 232.89316) -> (-65.918765, 229.645432) ccw
  ellipse E52 centre (-161.503857, 152.189905) end of major axis (-140.392474, 132.932695) minor radius 28.574691 (-134.342818, 143.312652) -> (-134.09856, 160.281098) ccw
  ellipse E53 centre (-161.503857, 152.189905) end of major axis (-140.392474, 132.932695) minor radius 28.574691 (-140.224424, 171.260796) -> (-152.260969, 179.228485) ccw
  ellipse E54 centre (56.860407, 274.019239) end of major axis (91.576902, 242.351827) minor radius 46.989492 (13.023166, 290.941123) -> (13.037254, 257.06185) ccw
  ellipse E55 centre (-134.806635, 175.083334) end of major axis (-137.152344, 177.223025) minor radius 3.174966 (-133.2597, 172.310683) -> (-131.963746, 176.496989) ccw
  ellipse E56 centre (-137.860042, 173.379784) end of major axis (-135.514333, 171.240094) minor radius 3.174966 (-140.224424, 171.260796) -> (-136.313107, 170.607133) ccw
  ellipse E57 centre (10.07623, 255.91608) end of major axis (7.730521, 258.05577) minor radius 3.174966 (11.623165, 253.143429) -> (13.037254, 257.06185) ccw
  ellipse E58 centre (3.563925, 252.282748) end of major axis (5.909634, 250.143058) minor radius 3.174966 (0.88147, 250.584261) -> (5.11086, 249.510097) ccw
  ellipse E59 centre (-30.765008, 181.835248) end of major axis (-33.110717, 183.974938) minor radius 3.174966 (-27.730197, 180.902237) -> (-28.591878, 184.149965) ccw
  ellipse E60 centre (-128.579407, 162.560475) end of major axis (-130.925117, 164.700165) minor radius 3.174966 (-125.736518, 163.974129) -> (-130.126343, 165.333126) ccw
  ellipse E61 centre (-131.053527, 161.180119) end of major axis (-133.399236, 163.319809) minor radius 3.174966 (-132.600462, 163.95277) -> (-134.09856, 160.281098) ccw
  ellipse E62 centre (16.882745, 243.716415) end of major axis (14.537036, 245.856105) minor radius 3.174966 (19.412977, 245.634315) -> (15.33581, 246.489066) ccw
  ellipse E63 centre (11.048952, 240.461637) end of major axis (13.394661, 238.321947) minor radius 3.174966 (9.502017, 243.234289) -> (8.366497, 238.76315) ccw
  ellipse E64 centre (-161.503857, 152.189905) end of major axis (-177.923821, 167.167736) minor radius 22.22476 (-174.014593, 170.559215) -> (-182.087177, 160.573001) ccw
  ellipse E65 centre (-171.630308, 170.262351) end of major axis (-172.803163, 171.332196) minor radius 1.587483 (-170.318223, 171.15596) -> (-172.523932, 171.574445) ccw
  ellipse E66 centre (-167.991476, 164.919513) end of major axis (-169.16433, 165.989358) minor radius 1.587483 (-167.270629, 163.505112) -> (-166.679391, 165.813122) ccw
  ellipse E67 centre (-161.503857, 152.189905) end of major axis (-152.12102, 143.631145) minor radius 12.699863 (-167.270629, 163.505112) -> (-170.267749, 161.381433) ccw
  ellipse E68 centre (-167.049131, 149.096097) end of major axis (-176.431968, 157.654858) minor radius 12.699863 (-170.267749, 161.381433) -> (-176.727188, 157.319552) ccw
  ellipse E69 centre (-179.146702, 159.375416) end of major axis (-181.492412, 161.515106) minor radius 3.174966 (-182.087177, 160.573001) -> (-176.727188, 157.319552) ccw
  ellipse E70 centre (-159.129682, 135.337557) end of major axis (-156.783973, 133.197867) minor radius 3.174966 (-156.123569, 136.359195) -> (-160.713572, 138.089265) ccw
  ellipse E71 centre (-156.385722, 132.197199) end of major axis (-155.212867, 131.127353) minor radius 1.587483 (-155.992019, 130.659298) -> (-154.882666, 132.708018) ccw
  ellipse E72 centre (-161.503857, 152.189905) end of major axis (-177.923821, 167.167736) minor radius 22.22476 (-165.181112, 130.2714) -> (-155.992019, 130.659298) ccw
  ellipse E73 centre (-164.65579, 133.402615) end of major axis (-167.001499, 135.542305) minor radius 3.174966 (-165.134458, 136.541312) -> (-165.181112, 130.2714) ccw
  ellipse E74 centre (-167.049131, 149.096097) end of major axis (-176.431968, 157.654858) minor radius 12.699863 (-165.134458, 136.541312) -> (-160.713572, 138.089265) ccw
  ellipse E75 centre (68.57103, 299.386335) end of major axis (82.645285, 286.548195) minor radius 19.049794 (55.098278, 312.85435) -> (52.266053, 309.237727) ccw
  ellipse E76 centre (49.548556, 310.879625) end of major axis (51.894265, 308.739935) minor radius 3.174966 (47.663549, 308.324795) -> (52.266053, 309.237727) ccw
  ellipse E77 centre (36.353503, 292.995817) end of major axis (50.427758, 280.157676) minor radius 19.049794 (47.663549, 308.324795) -> (43.665253, 310.586549) ccw
  ellipse E78 centre (44.883878, 313.518337) end of major axis (47.229587, 311.378647) minor radius 3.174966 (43.962607, 316.55673) -> (43.665253, 310.586549) ccw
  ellipse E79 centre (56.860407, 274.019239) end of major axis (89.700335, 244.063579) minor radius 44.449519 (52.544543, 318.259003) -> (43.962607, 316.55673) ccw
  ellipse E80 centre (52.852819, 315.099019) end of major axis (50.50711, 317.23871) minor radius 3.174966 (55.098278, 312.85435) -> (52.544543, 318.259003) ccw
  ellipse E81 centre (84.604874, 270.72039) end of major axis (98.679129, 257.882249) minor radius 19.049794 (93.250283, 287.695433) -> (88.935431, 289.271476) ccw
  ellipse E82 centre (89.657191, 292.363323) end of major axis (92.0029, 290.223633) minor radius 3.174966 (86.644882, 293.366611) -> (88.935431, 289.271476) ccw
  ellipse E83 centre (68.57103, 299.386335) end of major axis (82.645285, 286.548195) minor radius 19.049794 (86.644882, 293.366611) -> (87.560357, 297.868109) ccw
  ellipse E84 centre (90.725245, 297.615072) end of major axis (88.379536, 299.754762) minor radius 3.174966 (93.330232, 299.430136) -> (87.560357, 297.868109) ccw
  ellipse E85 centre (56.860407, 274.019239) end of major axis (89.700335, 244.063579) minor radius 44.449519 (97.601244, 291.794251) -> (93.330232, 299.430136) ccw
  ellipse E86 centre (94.691184, 290.524607) end of major axis (97.036893, 288.384917) minor radius 3.174966 (93.250283, 287.695433) -> (97.601244, 291.794251) ccw
  ellipse E87 centre (56.860407, 274.019239) end of major axis (89.700335, 244.063579) minor radius 44.449519 (88.404012, 242.701459) -> (92.297799, 247.186547) ccw
  ellipse E88 centre (84.225981, 242.999651) end of major axis (86.571691, 240.859961) minor radius 3.174966 (81.093242, 243.515892) -> (86.479096, 240.762666) ccw
  ellipse E89 centre (62.296807, 246.613342) end of major axis (76.371062, 233.775202) minor radius 19.049794 (81.093242, 243.515892) -> (81.278216, 248.227153) ccw
  ellipse E90 centre (84.441784, 248.496121) end of major axis (82.096075, 250.635811) minor radius 3.174966 (84.465083, 251.671017) -> (81.278216, 248.227153) ccw
  ellipse E91 centre (84.604874, 270.72039) end of major axis (98.679129, 257.882249) minor radius 19.049794 (84.465083, 251.671017) -> (89.029173, 252.191342) ccw
  ellipse E92 centre (89.766556, 249.103168) end of major axis (87.420847, 251.242858) minor radius 3.174966 (92.297799, 247.186547) -> (89.029173, 252.191342) ccw
  ellipse E93 centre (-86.321419, 186.864106) end of major axis (-85.383136, 186.00823) minor radius 1.269986
  ellipse E94 centre (-75.230871, 193.051722) end of major axis (-74.292587, 192.195846) minor radius 1.269986
  ellipse E95 centre (-92.509161, 197.95471) end of major axis (-91.570877, 197.098834) minor radius 1.269986
  ellipse E96 centre (-81.418612, 204.142326) end of major axis (-80.480328, 203.28645) minor radius 1.269986
  ellipse E97 centre (-105.122313, 201.533892) end of major axis (-107.468022, 203.673582) minor radius 3.174966 (-106.669248, 204.306543) -> (-107.89495, 199.986988) ccw
  ellipse E98 centre (-108.434312, 194.43727) end of major axis (-106.088602, 192.29758) minor radius 3.174966 (-109.815782, 191.578606) -> (-105.661674, 195.984174) ccw
  ellipse E99 centre (-82.940945, 221.180702) end of major axis (-85.286654, 223.320392) minor radius 3.174966 (-81.39401, 218.408051) -> (-79.828176, 221.806125) ccw
  ellipse E100 centre (-96.58205, 173.193858) end of major axis (-98.927759, 175.333548) minor radius 3.174966 (-93.809413, 174.740762) -> (-95.20058, 176.052523) ccw
  ellipse E101 centre (-89.900469, 174.251005) end of major axis (-92.246178, 176.390695) minor radius 3.174966 (-92.673106, 172.704101) -> (-88.469858, 171.416583) ccw
  ellipse E102 centre (-87.039248, 168.58216) end of major axis (-84.693539, 166.44247) minor radius 3.174966 (-85.657777, 171.440825) -> (-88.469858, 171.416583) ccw
  ellipse E103 centre (32.506845, 193.516409) end of major axis (41.889681, 184.957649) minor radius 12.699863 (41.945987, 202.012828) -> (31.126905, 206.141156) ccw
  ellipse E104 centre (-62.617719, 189.47254) end of major axis (-60.27201, 187.33285) minor radius 3.174966 (-61.070784, 186.699889) -> (-59.845082, 191.019444) ccw
  ellipse E105 centre (-66.246076, 209.008716) end of major axis (-63.900367, 206.869026) minor radius 3.174966 (-69.358845, 208.383293) -> (-69.018713, 207.461812) ccw
  ellipse E106 centre (-15.590955, 177.170192) end of major axis (-6.208119, 168.611431) minor radius 12.699863 (-27.730197, 180.902237) -> (-28.270559, 176.451958) ccw
  ellipse E107 centre (-61.036786, 183.083143) end of major axis (-63.382495, 185.222833) minor radius 3.174966 (-62.583721, 185.855794) -> (-64.149554, 182.45772) ccw
  ellipse E108 centre (-20.138271, 276.658888) end of major axis (-10.755434, 268.100128) minor radius 12.699863 (-9.31609, 270.012816) -> (-8.110838, 280.736657) ccw
  ellipse E109 centre (-15.590955, 177.170192) end of major axis (-14.652672, 176.314316) minor radius 1.269986
  ellipse E110 centre (-63.688755, 160.823974) end of major axis (-62.750471, 159.968098) minor radius 1.269986
  ellipse E111 centre (32.506845, 193.516409) end of major axis (33.445128, 192.660533) minor radius 1.269986
  ellipse E112 centre (-111.786555, 144.477757) end of major axis (-110.848271, 143.621881) minor radius 1.269986
  ellipse E113 centre (-20.138271, 276.658888) end of major axis (-21.076554, 277.514764) minor radius 1.269986
  ellipse E114 centre (84.604874, 270.72039) end of major axis (83.66659, 271.576266) minor radius 1.269986
  ellipse E115 centre (68.57103, 299.386335) end of major axis (67.632746, 300.242211) minor radius 1.269986
  ellipse E116 centre (-78.919688, 236.625205) end of major axis (-79.857971, 237.481081) minor radius 1.269986
  ellipse E117 centre (32.47582, 260.380313) end of major axis (31.537536, 261.236189) minor radius 1.269986
  ellipse E118 centre (62.296807, 246.613342) end of major axis (61.358524, 247.469218) minor radius 1.269986
  ellipse E119 centre (36.353503, 292.995817) end of major axis (35.415219, 293.851693) minor radius 1.269986
  ellipse E120 centre (-137.701105, 196.591521) end of major axis (-138.639388, 197.447397) minor radius 1.269986
  ellipse E121 centre (56.860407, 274.019239) end of major axis (46.539286, 283.433876) minor radius 13.969849
  ellipse E122 centre (-5.10398, 281.756099) end of major axis (-2.758271, 279.616409) minor radius 3.174966 (-6.891228, 284.380286) -> (-8.110838, 280.736657) ccw
  ellipse E123 centre (10.06119, 292.084493) end of major axis (7.715481, 294.224183) minor radius 3.174966 (13.023166, 290.941123) -> (8.273942, 294.70868) ccw
  ellipse E124 centre (-125.099314, 186.936965) end of major axis (-122.753605, 184.797275) minor radius 3.174966 (-127.619672, 188.867877) -> (-127.942203, 185.523311) ccw
  ellipse E125 centre (-125.077949, 186.964917) end of major axis (-122.73224, 184.825227) minor radius 3.174966 (-123.696478, 189.823582) -> (-127.60258, 188.890238) ccw
  ellipse E126 centre (-137.701105, 196.591521) end of major axis (-147.083941, 205.150282) minor radius 12.699863 (-127.619672, 188.867877) -> (-127.60258, 188.890238) ccw
  line L52 (-6.891228, 284.380286) -> (8.273942, 294.70868)
  point P0 (56.90893, 215.989808)
  point P1 (-10.954295, 193.903537)
  point P2 (-76.321337, 52.092718)
  point P3 (-102.010854, 140.78445)
  point P4 (-6.35, 163.875478)
  point P5 (-6.35, 113.075478)
  point P6 (-74.735, 212.838914)
  point P7 (-74.735, 212.838914)
  point P8 (-6.35, 113.075478)
  point P9 (-29.65, -33.116159)
  point P10 (-29.65, -33.116159)
  point P11 (-74.735, 212.838914)
  point P12 (-50.834886, 12.533639)
  point P13 (-50.854476, 12.562862)
  point P14 (-50.834886, 12.533639)
  point P15 (-50.854476, 12.562862)
  point P16 (-50.834886, 12.533639)
  point P17 (-50.854476, 12.562862)
  point P18 (-101.999257, 156.659446)
  point P19 (-106.89852, 174.341704)